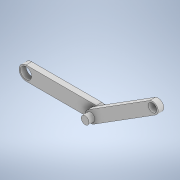
# Autodesk Inventor part: Part2
Saved by Autodesk Inventor 2021 (Build 250183000, 183)
## iProperties
Created: 2022-03-10
Part Number: Part2
Material: Generic
Document SubType Name: Modeling
Designer: User
Density: 1 g/cm^3
Appearance: Default
Author: User
Autodesk Inventor part; units mm, degrees
ref_plane "YZ Plane" through (0, 0, 0) normal (1, 0, 0) x (0, 1, 0)
ref_plane "XZ Plane" through (0, 0, 0) normal (0, 1, 0) x (-1, 0, 0)
ref_plane "XY Plane" through (0, 0, 0) normal (0, 0, 1) x (1, 0, 0)
sketch "Sketch1" plane through (0, 0, 0) normal (0, 0, 1) x (1, 0, 0)
  line L0 (-30.9725, 9.5014) -> (-0.9725, 9.5014) construction
  line L1 (-28.4725, 7.0014) -> (-3.4725, 7.0014)
  line L2 (-3.4725, 12.0014) -> (-28.4725, 12.0014)
  arc A0 (-28.4725, 12.0014) -> (-28.4725, 7.0014) centre (-28.4725, 9.5014) ccw
  arc A1 (-3.4725, 7.0014) -> (-3.4725, 12.0014) centre (-3.4725, 9.5014) ccw
  circle A2 centre (-28.4725, 9.5014) radius 2
  circle A3 centre (-3.4725, 9.5014) radius 2
  point P0 (0, 0)
  point P1 (-15.9725, 9.5014)
  dimension "d0" = 30
  dimension "d1" = 5
  dimension "d2" = 4
  dimension "d3" = 4
  constraints: 8 end point, 6 point on circle, 4 centre point, 4 tangent, 2 coincident, 2 point on line, 1 horizontal, 1 midpoint, 1 parallel
  measures "d0" distance of L0.start L0.end
  measures "d1" diameter of A1
  measures "d2" diameter of A2
  measures "d3" diameter of A3
sketch "Sketch2" plane through (0, 0, 0) normal (0, 0, 1) x (1, 0, 0)
  line L0 (-5.1503, 8.4208) -> (20.2439, 24.3938) construction
  line L1 (-2.3925, 7.7927) -> (19.6158, 21.636)
  line L2 (17.486, 25.0219) -> (-4.5222, 11.1786)
  arc A0 (-4.5222, 11.1786) -> (-2.3925, 7.7927) centre (-3.4574, 9.4857) ccw
  arc A1 (19.6158, 21.636) -> (17.486, 25.0219) centre (18.5509, 23.3289) ccw
  circle A2 centre (18.5509, 23.3289) radius 1.5
  circle A3 centre (-3.4574, 9.4857) radius 1.5
  circle A4 centre (-3.4574, 9.4857) radius 1.5
  point P0 (0, 0)
  point P1 (7.5468, 16.4073)
  dimension "d4" = 30
  dimension "d5" = 4
  dimension "d6" = 3
  dimension "d9" = 3
  dimension "d12" = 3
  constraints: 8 end point, 6 point on circle, 5 centre point, 4 tangent, 3 coincident, 2 point on line, 1 midpoint, 1 parallel
  measures "d4" distance of L0.start L0.end
  measures "d5" diameter of A1
  measures "d6" diameter of A2
  measures "d9" diameter of A3
  measures "d12" diameter of A4
extrude "Extrusion1" add sketch "Sketch1" against normal blind 2
extrude "Extrusion2" add sketch "Sketch2" along normal blind 2
sketch "Sketch5" plane through (0, 0, 2) normal (0, 0, 1) x (1, 0, 0)
  circle A0 centre (-3.4574, 9.4857) radius 1.4
  circle A1 centre (-3.4574, 9.4857) radius 1.5 projected
  point P0 (0, 0)
  dimension "d13" = 2.8
  constraints: 1 centre point, 1 concentric
  measures "d13" diameter of A0
extrude "Extrusion3" add sketch "Sketch5" along normal blind 2 and the other way blind 5 contours A0
body "Solid1"
